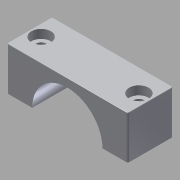
# Autodesk Inventor part: 2.5 CIM mount
Saved by Autodesk Inventor 2013 (Build 170138000, 138)
## iProperties
Created: 2013-01-18
Part Number: 2.5 CIM mount
Material: ABS Plastic
Document SubType Name: Modeling
Designer: Naphat
Density: 1 g/cm^3
Author: Naphat
Autodesk Inventor part; units mm, degrees
ref_plane "YZ Plane" through (0, 0, 0) normal (1, 0, 0) x (0, 1, 0)
ref_plane "XZ Plane" through (0, 0, 0) normal (0, 1, 0) x (-1, 0, 0)
ref_plane "XY Plane" through (0, 0, 0) normal (0, 0, 1) x (1, 0, 0)
sketch "Sketch2" plane through (0, 0, 0) normal (0, 1, 0) x (-1, 0, 0)
  line L0 (-15.2041, -8.8425) -> (269.2759, -8.8425)
  line L1 (269.2759, -8.8425) -> (269.2759, 97.8375)
  line L2 (269.2759, 97.8375) -> (-15.2041, 97.8375)
  line L3 (-15.2041, 97.8375) -> (-15.2041, -8.8425)
  point P0 (0, 0)
  dimension "d5" = 284.48
  dimension "d6" = 106.68
  dimension "d7" = 284.48
  dimension "d8" = 106.68
  constraints: 8 end point, 1 horizontal, 1 parallel, 1 perpendicular
  measures "d5" distance of L0.start L0.end
  measures "d6" distance of L0.end L1.end
  measures "d7" distance of L1.end L2.end
  measures "d8" distance of L2.end L0.start
extrude "Extrusion1" add sketch "Sketch2" along normal blind 101.6
sketch "Sketch3" plane through (15.2041, 0, -8.8425) normal (0, 0, -1) x (-1, 0, 0)
  line L0 (0, 0) -> (284.48, 0) projected
  arc A0 (224.79, 0) -> (59.69, 0) centre (142.24, 0) ccw
  line L1 (59.69, 0) -> (224.79, 0)
  point P0 (15.2041, 0)
  constraints: 2 end point, 2 point on circle, 2 point on line, 1 centre point, 1 collinear, 1 midpoint
extrude "Extrusion2" cut sketch "Sketch3" against normal blind 127
sketch "Sketch4" plane through (0, 0, 0) normal (0, -1, 0) x (1, 0, 0)
  line L0 (-209.5859, -8.8425) -> (-209.5859, 97.8375) projected
  line L1 (-269.2759, 97.8375) -> (-209.5859, 97.8375) projected
  line L2 (-269.2759, -8.8425) -> (-269.2759, 97.8375) projected
  line L3 (-209.5859, -8.8425) -> (-269.2759, -8.8425) projected
  line L4 (-44.4859, 97.8375) -> (15.2041, 97.8375) projected
  line L5 (-44.4859, 97.8375) -> (-44.4859, -8.8425) projected
  line L6 (15.2041, -8.8425) -> (-44.4859, -8.8425) projected
  line L7 (15.2041, 97.8375) -> (15.2041, -8.8425) projected
  line L8 (-44.4859, 97.8375) -> (15.2041, 97.8375) projected
  line L9 (-241.3709, 97.8375) -> (-241.3709, 91.4875) construction
  line L10 (-209.5859, 77.888) -> (-224.8259, 77.888) construction
  line L11 (-269.2759, 47.5596) -> (-259.1159, 47.5596) construction
  line L12 (-239.4309, -8.8425) -> (-239.4309, -2.4925) construction
  line L13 (-259.1159, -2.4925) -> (-259.1159, 91.4875)
  line L14 (-259.1159, 91.4875) -> (-224.8259, 91.4875)
  line L15 (-224.8259, 91.4875) -> (-224.8259, -2.4925)
  line L16 (-224.8259, -2.4925) -> (-259.1159, -2.4925)
  point P0 (0, 0)
  dimension "d15" = 6.35
  dimension "d16" = 15.24
  dimension "d17" = 10.16
  dimension "d18" = 6.35
  constraints: 16 end point, 6 perpendicular, 3 point on line, 1 midpoint, 1 parallel
  measures "d15" distance of L9.start L9.end
  measures "d16" distance of L10.start L10.end
  measures "d17" distance of L11.start L11.end
  measures "d18" distance of L12.start L12.end
extrude "Extrusion3" cut sketch "Sketch4" against normal blind 76.2 contours L13 L14 L15 L16
sketch "Sketch5" plane through (0, 76.2, 0) normal (0, -1, 0) x (1, 0, 0)
  line L0 (-259.1159, 91.4875) -> (-224.8259, 91.4875) projected
  line L1 (-259.1159, -2.4925) -> (-259.1159, 91.4875) projected
  line L2 (-224.8259, -2.4925) -> (-259.1159, -2.4925) projected
  line L3 (-224.8259, 91.4875) -> (-224.8259, -2.4925) projected
  line L4 (-259.1159, 44.4975) -> (-224.8259, 44.4975) construction
  line L5 (-241.9709, 91.4875) -> (-241.9709, 84.1907) construction
  line L6 (-241.9709, 84.1907) -> (-241.9709, 84.1907) construction
  line L7 (-241.9709, 84.1907) -> (-241.9709, -2.4925) construction
  circle A0 centre (-241.9709, 44.4975) radius 20.32
  point P0 (0, 0)
  dimension "d21" = 40.64
  dimension "d22" = 0
  constraints: 8 end point, 5 midpoint, 3 perpendicular, 1 centre point, 1 point on line
  measures "d21" diameter of A0
  measures "d22" distance of L5.end L6.end
extrude "Extrusion4" add sketch "Sketch5" along normal blind 76.2 contours A0 L3 L1 | L1 A0 | A0 L3
sketch "Sketch6" plane through (0, 0, 0) normal (0, -1, 0) x (1, 0, 0)
  arc A0 (-259.1159, 33.5911) -> (-224.8259, 33.5911) centre (-241.9709, 44.4975) ccw projected
  circle A1 centre (-241.9709, 44.4975) radius 12.7
  point P0 (0, 0)
  dimension "d25" = 25.4
  constraints: 1 centre point, 1 coincident
  measures "d25" diameter of A1
extrude "Extrusion5" cut sketch "Sketch6" against normal blind 101.6
sketch "Sketch7" plane through (0, 101.6, 0) normal (0, 1, 0) x (1, 0, 0)
  circle A0 centre (-241.9709, -44.4975) radius 12.7 projected
  circle A1 centre (-241.9709, -44.4975) radius 22.86
  point P0 (0, 0)
  dimension "d29" = 45.72
  constraints: 1 centre point, 1 coincident
  measures "d29" diameter of A1
extrude "Extrusion6" cut sketch "Sketch7" against normal blind 20.32
sketch "Sketch8" plane through (0, 0, 0) normal (0, -1, 0) x (1, 0, 0)
  line L0 (-44.4859, 97.8375) -> (-44.4859, -8.8425) projected
  line L1 (15.2041, -8.8425) -> (-44.4859, -8.8425) projected
  line L2 (15.2041, 97.8375) -> (15.2041, -8.8425) projected
  line L3 (-44.4859, 97.8375) -> (15.2041, 97.8375) projected
  line L4 (-44.4859, 51.8911) -> (-29.2459, 51.8911) construction
  line L5 (15.2041, 49.6514) -> (5.0441, 49.6514) construction
  line L6 (-16.6435, -8.8425) -> (-16.6435, -2.4925) construction
  line L7 (-14.6409, 97.8375) -> (-14.6409, 91.4875) construction
  line L8 (5.0441, 91.4875) -> (-29.2459, 91.4875)
  line L9 (-29.2459, 91.4875) -> (-29.2459, -2.4925)
  line L10 (-29.2459, -2.4925) -> (5.0441, -2.4925)
  line L11 (5.0441, -2.4925) -> (5.0441, 91.4875)
  point P0 (0, 0)
  dimension "d32" = 15.24
  dimension "d33" = 10.16
  dimension "d34" = 6.35
  dimension "d35" = 6.35
  constraints: 16 end point, 4 parallel, 4 perpendicular, 3 point on line, 1 midpoint
  measures "d32" distance of L4.start L4.end
  measures "d33" distance of L5.start L5.end
  measures "d34" distance of L6.start L6.end
  measures "d35" distance of L7.start L7.end
extrude "Extrusion7" cut sketch "Sketch8" against normal blind 76.2 contours L11 L10 L9 L8
sketch "Sketch9" plane through (0, 76.2, 0) normal (0, -1, 0) x (1, 0, 0)
  line L0 (-29.2459, 91.4875) -> (5.0441, 91.4875) projected
  line L1 (-29.2459, -2.4925) -> (-29.2459, 91.4875) projected
  line L2 (5.0441, -2.4925) -> (-29.2459, -2.4925) projected
  line L3 (-12.1009, -2.4925) -> (-12.1009, 91.4875) construction
  line L4 (-29.2459, 44.4975) -> (0, 44.4975) construction
  circle A0 centre (-12.1009, 44.4975) radius 20.32
  point P0 (0, 0)
  dimension "d38" = 40.64
  constraints: 4 end point, 4 midpoint, 1 centre point, 1 perpendicular, 1 point on line
  measures "d38" diameter of A0
extrude "Extrusion8" add sketch "Sketch9" along normal blind 76.2
sketch "Sketch10" plane through (0, 0, 0) normal (0, -1, 0) x (1, 0, 0)
  arc A0 (-29.2459, 33.5911) -> (5.0441, 33.5911) centre (-12.1009, 44.4975) ccw projected
  circle A1 centre (-12.1009, 44.4975) radius 12.7
  point P0 (0, 0)
  dimension "d41" = 25.4
  constraints: 1 centre point, 1 coincident
  measures "d41" diameter of A1
extrude "Extrusion9" cut sketch "Sketch10" against normal blind 101.6
sketch "Sketch11" plane through (0, 101.6, 0) normal (0, 1, 0) x (1, 0, 0)
  circle A0 centre (-12.1009, -44.4975) radius 12.7 projected
  circle A1 centre (-12.1009, -44.4975) radius 22.86
  point P0 (0, 0)
  dimension "d44" = 45.72
  constraints: 1 centre point, 1 coincident
  measures "d44" diameter of A1
extrude "Extrusion10" cut sketch "Sketch11" against normal blind 20.32
fillet "Fillet1" radius 4 4 edges at (15.2041, 50.8, 97.8375) (15.2041, 50.8, -8.8425) (-269.2759, 50.8, 97.8375) (-269.2759, 50.8, -8.8425)
fillet "Fillet2" radius 1 8 edges at (14.0325, 101.6, 96.666) (15.2041, 101.6, 44.4975) (14.0325, 101.6, -7.6709) (-127.0359, 101.6, -8.8425) (-268.1044, 101.6, -7.6709) (-269.2759, 101.6, 44.4975) (-268.1044, 101.6, 96.666) (-127.0359, 101.6, 97.8375)
body "Solid1"
